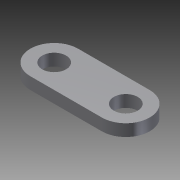
# Autodesk Inventor part: lesson3
Saved by Autodesk Inventor 2011 SP1 (Build 150282100, 282)
## iProperties
Created: 2011-10-07
Part Number: lesson3
Document SubType Name: Modeling
Designer: Kevin
Density: 1 g/cm^3
Author: Kevin
Autodesk Inventor part; units mm, degrees
ref_plane "YZ Plane" through (0, 0, 0) normal (1, 0, 0) x (0, 1, 0)
ref_plane "XZ Plane" through (0, 0, 0) normal (0, 1, 0) x (-1, 0, 0)
ref_plane "XY Plane" through (0, 0, 0) normal (0, 0, 1) x (1, 0, 0)
sketch "Sketch1" plane through (0, 0, 0) normal (0, 0, 1) x (1, 0, 0)
  arc A0 (-13.1138, 9.0719) -> (-13.1138, -10.9281) centre (-13.1138, -0.9281) ccw
  arc A1 (16.8862, -10.9281) -> (16.8862, 9.0719) centre (16.8862, -0.9281) ccw
  line L0 (-13.1138, 9.0719) -> (16.8862, 9.0719)
  line L1 (-13.1138, -10.9281) -> (16.8862, -10.9281)
  circle A2 centre (-13.1138, -0.9281) radius 5
  circle A3 centre (16.8862, -0.9281) radius 5
  point P0 (0, 0)
  dimension "d0" = 20
  dimension "d1" = 20
  dimension "d2" = 30
  dimension "d3" = 10
  dimension "d4" = 10
  constraints: 4 centre point, 4 end point, 4 point on circle, 2 coincident, 2 tangent, 1 horizontal alignment, 1 parallel
  measures "d0" diameter of A0
  measures "d1" diameter of A1
  measures "d2" distance of L0.start L0.end
  measures "d3" diameter of A2
  measures "d4" diameter of A3
extrude "Extrusion1" add sketch "Sketch1" along normal blind 5
body "Solid1"
